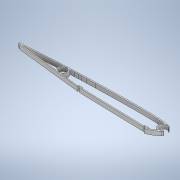
# Autodesk Inventor part: airfoil
Saved by Autodesk Inventor 2022 (Build 260153000, 153)
## iProperties
Created: 2021-03-06
Part Number: airfoil
Material: Generic
Document SubType Name: Modeling
Designer: Ferdinand Hubbard
Density: 1 g/cm^3
Appearance: Default
Author: Ferdinand Hubbard
Autodesk Inventor part; units mm, degrees
ref_plane "YZ Plane" through (0, 0, 0) normal (1, 0, 0) x (0, 1, 0)
ref_plane "XZ Plane" through (0, 0, 0) normal (0, 1, 0) x (-1, 0, 0)
ref_plane "XY Plane" through (0, 0, 0) normal (0, 0, 1) x (1, 0, 0)
sketch "Sketch1" plane through (0, 0, 0) normal (0, 1, 0) x (-1, 0, 0)
  line L0 (211.8455, 21.5812) -> (210.9592, -8.8383) construction
  circle A0 centre (258.2615, 4.8535) radius 8
  spline S0 degree 4 poles (34.5603, 29.5437) (33.7959, 29.2698) (30.8112, 28.1631) (25.9991, 26.1225) (19.6138, 22.8804) (11.2549, 17.3272) (6.0635, 12.605) (2.8423, 8.0332) (1.9781, 6.5051) knots 0.291118 0.291118 0.291118 0.291118 0.291118 0.338648 0.479254 0.612645 0.738339 1 1 1 1 1
  line L1 (229.1022, 19.6309) -> (363.9286, 4.3933)
  circle A1 centre (370.8333, 3.6129) radius 4 construction
  spline S1 degree 4 poles (6.5182, -5.2336) (7.1494, -5.5885) (14.4657, -7.5137) (22.7137, -8.712) (35.9318, -9.9587) (48.9047, -10.4891) (62.2875, -10.9022) (78.073, -11.0572) (94.7047, -11.0677) (112.5814, -10.9206) (131.2146, -10.6478) (157.2989, -10.1249) (178.3611, -9.5706) (196.5094, -9.0102) (204.4618, -8.7595) knots 0 0 0 0 0 0.111054 0.172284 0.238398 0.309093 0.3838 0.461605 0.542502 0.625628 0.710437 0.796395 1 1 1 1 1
  arc A2 (204.8781, 22.3686) -> (204.3228, 22.4313) centre (203.7026, 14.4554) ccw
  line L2 (204.4618, -8.7595) -> (204.4618, -8.7595) construction
  arc A3 (204.4618, -8.7595) -> (204.4618, -8.7595) centre (-110.5763, 9986.2768) ccw construction
  line L3 (204.3228, 22.4313) -> (205.1008, 22.3434)
  arc A4 (366.8584, 4.0604) -> (366.7756, 4.0715) centre (366.551, 2.0842) ccw
  line L4 (205.1008, 22.3434) -> (229.1022, 19.6309)
  line L5 (204.4618, -8.7595) -> (226.4407, -8.0668)
  circle A5 centre (13.7691, 4.0715) radius 9.5
  circle A6 centre (13.7691, 4.0715) radius 8
  line L6 (6.5181, 10.2093) -> (6.4686, 10.2474)
  line L7 (6.5181, -2.0663) -> (6.4883, -2.0926)
  line L8 (6.3756, -3.4733) -> (8.2772, -5.8071)
  line L9 (6.2475, 11.5973) -> (7.6237, 13.6489)
  line L10 (7.6236, 9.1933) -> (7.4154, 9.3611)
  line L11 (7.111, 10.5032) -> (8.7725, 14.7639)
  line L12 (7.7077, -1.1495) -> (7.655, -1.1924)
  line L13 (7.6239, -2.4061) -> (12.536, -6.8462)
  arc A7 (6.4883, -2.0926) -> (6.3756, -3.4733) centre (7.1509, -2.8416) ccw
  arc A8 (7.655, -1.1924) -> (7.6239, -2.4061) centre (8.1603, -1.8126) ccw
  arc A9 (7.111, 10.5032) -> (7.4154, 9.3611) centre (8.0427, 10.1399) ccw
  arc A10 (6.2475, 11.5973) -> (6.4686, 10.2474) centre (7.078, 11.0402) ccw
  circle A11 centre (258.2615, 4.8535) radius 9.5
  line L14 (199.7021, 25.262) -> (204.7021, 25.262)
  line L15 (204.7021, 25.262) -> (204.7021, 20.262)
  line L16 (204.7021, 20.262) -> (199.7021, 20.262)
  line L17 (199.7021, 20.262) -> (199.7021, 25.262)
  line L18 (363.9286, 7.3389) -> (368.9286, 7.3389)
  line L19 (368.9286, 7.3389) -> (368.9286, 2.3389)
  line L20 (368.9286, 2.3389) -> (363.9286, 2.3389)
  line L21 (363.9286, 2.3389) -> (363.9286, 7.3389)
  line L22 (368.9286, 2.3389) -> (368.9286, 1.9316)
  arc A12 (366.9727, -0.0679) -> (368.9286, 1.9316) centre (366.9286, 1.9316) ccw
  spline S2 degree 4 poles (226.4407, -8.0668) (226.7168, -7.9106) (246.397, -7.271) (261.9174, -6.5757) (283.9748, -5.5203) (299.9172, -4.5963) (314.7263, -3.6143) (328.2274, -2.6448) (339.6733, -1.7771) (350.204, -1.0417) (357.3568, -0.5279) (364.7416, -0.1778) (365.8834, -0.1194) (366.8566, -0.0835) knots 0 0 0 0 0 0.209603 0.316305 0.419804 0.519462 0.614592 0.704374 0.787764 0.863385 0.925581 1 1 1 1 1
  spline S3 degree 4 poles (369.983, -0.0016) (369.9988, -0.0007) (370.0055, 0.0002) (370.0019, 0.001) (369.9872, 0.0018) knots 0 0 0 0 0 1 1 1 1 1
  line L23 (369.9445, -0.0037) -> (370.0215, 0.0006) construction
  arc A13 (369.9522, -0.0026) -> (370.0137, 0.0008) centre (369.9433, 0.7095) ccw construction
  line L24 (366.9727, -0.0679) -> (366.8566, -0.0835)
  line L25 (34.5603, 29.6339) -> (39.5603, 29.6339)
  line L26 (39.5603, 29.6339) -> (39.5603, 24.6339)
  line L27 (39.5603, 24.6339) -> (34.5603, 24.6339)
  line L28 (34.5603, 24.6339) -> (34.5603, 29.6339)
  line L29 (204.3228, 22.4313) -> (39.5603, 26.8701)
  line L30 (40.7281, 31.7535) -> (28.3924, 27.3339) construction
  arc A14 (39.5344, 31.1784) -> (29.6797, 27.6477) centre (67.8642, -63.4133) ccw construction
  arc A15 (16.4455, -7.6262) -> (9.219, 15.1754) centre (13.7691, 4.0715) ccw
  spline S4 degree 3 poles (31.9917, 25.5945) (29.42, 24.6117) (18.9132, 19.5206) (14.8641, 16.0215) knots 0 0 0 0 1 1 1 1
  line L31 (39.5603, 22.1339) -> (34.5603, 22.1339)
  line L32 (31.9917, 25.5945) -> (31.9917, 22.1339)
  line L33 (31.9917, 22.1339) -> (34.5603, 22.1339)
  line L34 (39.5603, 22.1339) -> (42.0603, 22.1339)
  line L35 (199.7021, 17.762) -> (204.7021, 17.762)
  line L36 (42.0603, 24.3027) -> (42.0603, 22.1339)
  line L37 (197.2021, 20.262) -> (197.2021, 17.762)
  line L38 (197.2021, 17.762) -> (207.2021, 17.762)
  line L39 (42.0603, 24.3027) -> (197.2021, 20.262)
  line L40 (207.2021, 17.762) -> (207.2021, 20.262)
  line L41 (207.2021, 20.262) -> (361.2547, 2.3389)
  line L42 (361.2547, 2.3389) -> (361.2518, 2.3349)
  spline S5 degree 2 poles (222.1769, -5.5406) (224.1126, -5.4289) (230.6005, -5.2002) knots 0 0 0 1 1 1
  spline S6 degree 2 poles (238.7466, -4.8781) (243.1919, -4.7074) (255.3149, -4.178) knots 0 0 0 1 1 1
  spline S7 degree 4 poles (262.0042, -3.8782) (272.1918, -3.4054) (286.4955, -2.6821) (303.5524, -1.5974) (322.555, -0.2289) (334.227, 0.6468) (346.6813, 1.5372) (354.3185, 2.0396) (360.4115, 2.3022) (361.2518, 2.3349) knots 0 0 0 0 0 0.344709 0.474433 0.596866 0.710582 0.813704 1 1 1 1 1
  line L43 (210.3278, -5.914) -> (222.1769, -5.5406)
  spline S8 degree 4 poles (21.2322, -5.3254) (22.7398, -5.5868) (33.0482, -6.8575) (45.691, -7.369) (62.6715, -7.9139) (78.3456, -8.0584) (95.0262, -8.0731) (112.874, -7.9246) (138.7995, -7.5451) (160.768, -7.0475) (178.0664, -6.5767) (190.4795, -6.2029) knots 0 0 0 0 0 0.165965 0.251662 0.34222 0.436535 0.534597 0.635362 0.738166 1 1 1 1 1
  arc A16 (251.9449, 15.0564) -> (250.6005, -4.3828) centre (258.2615, 4.8535) ccw
  arc A17 (266.723, -3.6555) -> (266.7518, 13.3337) centre (258.2615, 4.8535) ccw
  line L44 (190.4795, -6.2029) -> (210.3278, -5.914)
  line L45 (230.6005, -5.2002) -> (238.7466, -4.8781)
  point P0 (0, 0)
  point P1 (35.937, 30.0257)
  point P2 (12.8156, 18.139)
  point P3 (3.7499, 9.1521)
  point P4 (1.2115, 4.8535)
  point P5 (0.0668, 1.0195)
  point P6 (0.0003, -0.0638)
  point P7 (0.0755, -0.9849)
  point P8 (0.2106, -1.5356)
  point P9 (0.4302, -2.0122)
  point P10 (0.7739, -2.4345)
  point P11 (1.2488, -2.8423)
  point P12 (2.1566, -3.4383)
  point P13 (3.2773, -4.0196)
  point P14 (15.3669, -7.4261)
  point P15 (24.3167, -8.7706)
  point P16 (35.0526, -9.7678)
  point P17 (47.9909, -10.4262)
  point P18 (61.6814, -10.8267)
  point P19 (77.2847, -11.0213)
  point P20 (94.162, -11.0379)
  point P21 (112.1091, -10.9014)
  point P22 (130.911, -10.6315)
  point P23 (150.3435, -10.2474)
  point P24 (170.176, -9.7646)
  point P25 (190.1737, -9.1986)
  point P26 (248.7963, -7.1166)
  point P27 (267.1071, -6.3194)
  point P28 (284.4371, -5.4606)
  point P29 (300.619, -4.5258)
  point P30 (315.5184, -3.5432)
  point P31 (328.988, -2.5786)
  point P32 (340.8625, -1.7041)
  point P33 (350.9622, -0.9861)
  point P34 (359.0984, -0.4682)
  point P35 (365.0855, -0.1602)
  point P36 (368.7597, -0.0285)
  point P37 (112.1091, -11.9485)
  point P38 (1.9781, 6.5051)
  point P39 (370.8333, 3.6129)
  point P40 (204.4618, -8.7595)
  point P41 (5.7252, 10.8187)
  point P42 (5.7691, -2.7289)
  point P43 (6.8449, 9.8206)
  point P44 (6.9324, -1.7811)
  point P45 (46.0163, 32.9548)
  point P46 (369.983, -0.0016)
  point P47 (34.5603, 29.5437)
  point P48 (14.8641, 16.0215)
  point P49 (261.5022, -3.9011)
  point P50 (295.0142, -2.1075)
  point P51 (309.9136, -1.1249)
  point P52 (323.3832, -0.1603)
  point P53 (335.2577, 0.7142)
  point P54 (345.3574, 1.4323)
  point P55 (353.4935, 1.9502)
  point P56 (359.4807, 2.2581)
  point P57 (255.3149, -4.178)
  point P58 (8.583, -2.8113)
  point P59 (15.6728, -4.4303)
  point P60 (48.2968, -7.4304)
  point P61 (61.9872, -7.8309)
  point P62 (77.5905, -8.0255)
  point P63 (94.4679, -8.0421)
  point P64 (112.415, -7.9056)
  point P65 (131.2168, -7.6358)
  point P66 (150.6493, -7.2516)
  point P67 (170.4819, -6.7688)
  point P68 (21.2322, -5.3254)
  point P69 (21.2322, -5.3254)
  point P70 (21.2322, -5.3254)
  point P71 (204.4618, -8.7595)
  point P72 (204.7021, 22.3885)
  point P73 (199.7021, 22.5558)
  point P74 (222.1769, -5.5406)
  dimension "d69" = 8
  dimension "d50" = 368.7594
  dimension "d57" = 16
  dimension "d80" = 19
  dimension "d81" = 16
  dimension "d82" = 1
  dimension "d83" = 1
  dimension "d84" = 1
  dimension "d85" = 1
  dimension "d86" = 1
  dimension "d87" = 0.8
  dimension "d88" = 1
  dimension "d90" = 19
  dimension "d94" = 5
  dimension "d95" = 5
  dimension "d105" = 5
  dimension "d106" = 5
  dimension "d108" = 2
  dimension "d114" = 5
  dimension "d115" = 5
  dimension "d116" = 24
  dimension "d117" = 2.5
  dimension "d118" = 2.5
  dimension "d123" = 2.5
  dimension "d124" = 2.5
  dimension "d125" = 10
  constraints: 92 end point, 31 point on circle, 17 centre point, 16 point on line, 10 tangent, 6 midpoint, 6 parallel, 5 coincident, 4 horizontal, 3 perpendicular, 3 vertical, 2 collinear, 1 equal radius, 87 other
  measures "d50" distance of point (368.76, -0.028) point (0, -0.064)
  measures "d57" diameter of A0
  measures "d80" diameter of A5
  measures "d81" diameter of A6
  measures "d82" distance of L6.start point (5.725, 10.819)
  measures "d83" distance of L7.start point (5.769, -2.729)
  measures "d84" distance of L10.start point (6.845, 9.821)
  measures "d85" distance of L12.start point (6.932, -1.781)
  measures "d86" radius of A7
  measures "d87" radius of A8
  measures "d88" radius of A9
  measures "d90" diameter of A11
  measures "d94" distance of L15.end L16.end
  measures "d95" distance of L14.end L15.end
  measures "d105" distance of L19.end L20.end
  measures "d106" distance of L18.end L19.end
  measures "d108" radius of A12
  measures "d114" distance of L26.end L27.end
  measures "d115" distance of L25.end L26.end
  measures "d116" diameter of A15
  measures "d117" distance of L26.end L31.start
  measures "d118" distance of L31.start L34.end
  measures "d123" distance of L16.end L37.start
  measures "d124" distance of L37.start L37.end
  measures "d125" distance of L37.end L38.end
extrude "Extrusion5" add sketch "Sketch1" along normal blind 10 contours L28 L27 L26 L29 L17 L16 L15 A2 L3 L4 L1 L21 L20 L22 A12 L24 S2 L5 S1 A15 S8 L44 L43 S5 L45 S6 A11 S7 L42 L41 L40 L38 L35 L37 L39 L36 L34 L31 L33 L32 S4 S0 | A15 S1 L13 A5 L11 S0 | L11 A5 L6 A10 L9 S0 | L13 S1 L8 A7 L7 A5 | A16 L41 A11 S6 | A11 L41 A17 S7
body "Solid5"
